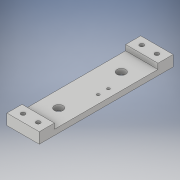
# Autodesk Inventor part: joint1_gear_holder
Saved by Autodesk Inventor 2019 (Build 230136000, 136)
## iProperties
Created: 2019-12-26
Part Number: joint1_gear_holder
Material: Типовые
Document SubType Name: Modeling
Designer: Петров Иван
Density: 1 g/cm^3
Appearance: По умолчанию
Author: Петров Иван
Autodesk Inventor part; units mm, degrees
ref_plane "YZ Plane" through (0, 0, 0) normal (1, 0, 0) x (0, 1, 0)
ref_plane "XZ Plane" through (0, 0, 0) normal (0, 1, 0) x (-1, 0, 0)
ref_plane "XY Plane" through (0, 0, 0) normal (0, 0, 1) x (1, 0, 0)
sketch "Эскиз1" plane through (0, 0, 0) normal (0, 1, 0) x (-1, 0, 0)
  line L0 (-15, 62) -> (15, 62)
  line L1 (15, 62) -> (15, -62)
  line L2 (15, -62) -> (-15, -62)
  line L3 (-15, -62) -> (-15, 62)
  line L4 (-15, 62) -> (15, -62) construction
  line L5 (15, 62) -> (-15, -62) construction
  point P0 (0, 0)
  dimension "d0" = 30
  dimension "d1" = 124
  constraints: 12 end point, 2 midpoint, 2 parallel, 1 horizontal, 1 perpendicular
  measures "d0" distance of L1.end L2.end
  measures "d1" distance of L0.end L1.end
extrude "Выдавливание1" add sketch "Эскиз1" along normal blind 5
sketch "Эскиз2" plane through (0, 5, 0) normal (0, 1, 0) x (1, 0, 0)
  line L0 (-15, -62) -> (15, -62) projected
  line L1 (15, -62) -> (15, 62) projected
  line L2 (-15, -62) -> (15, -62)
  line L3 (15, -62) -> (15, -48)
  line L4 (15, -48) -> (-15, -48)
  line L5 (-15, -48) -> (-15, -62)
  point P0 (0, 0)
  dimension "d4" = 14
  constraints: 8 end point, 2 parallel, 1 horizontal, 1 perpendicular, 1 point on line
  measures "d4" distance of L3.end L2.end
extrude "Выдавливание2" add sketch "Эскиз2" along normal blind 5
mirror "Зеркальное отражение1" about plane through (0, 0, 0) normal (0, 0, 1) of "Выдавливание2"
sketch "Эскиз3" plane through (0, 5, 0) normal (0, 1, 0) x (1, 0, 0)
  line L0 (15, 48) -> (-15, 48) projected
  line L1 (0, 48) -> (0, 29)
  circle A0 centre (0, 29) radius 4
  point P0 (0, 0)
  dimension "d7" = 19
  dimension "d8" = 8
  constraints: 2 end point, 1 centre point, 1 coincident, 1 midpoint, 1 vertical
  measures "d7" distance of L1.start L1.end
  measures "d8" diameter of A0
extrude "Выдавливание3" cut sketch "Эскиз3" against normal blind 15
mirror "Зеркальное отражение2" about plane through (0, 0, 0) normal (0, 0, 1) of "Выдавливание3"
sketch "Эскиз4" plane through (0, 0, 0) normal (0, -1, 0) x (1, 0, 0)
  line L0 (15, -62) -> (15, 62) projected
  line L1 (15, 48) -> (-15, 48) projected
  line L2 (15, 62) -> (-15, 62)
  line L3 (-15, 62) -> (-15, 48)
  line L4 (-15, 48) -> (15, 48)
  line L5 (15, 48) -> (15, 62)
  line L6 (15, 62) -> (-15, 62) projected
  line L7 (0, 62) -> (0, 55)
  line L8 (0, 55) -> (7, 55)
  circle A0 centre (7, 55) radius 1.9
  circle A1 centre (-7, 55) radius 1.9
  point P0 (0, 0)
  dimension "d11" = 7
  dimension "d12" = 7
  dimension "d13" = 3.8
  constraints: 12 end point, 2 centre point, 2 parallel, 2 perpendicular, 1 coincident, 1 horizontal, 1 midpoint, 1 symmetric about line, 1 vertical, 1 other
  measures "d11" distance of L7.start L7.end
  measures "d12" distance of L7.end L8.end
  measures "d13" diameter of A0
extrude "Выдавливание4" cut sketch "Эскиз4" against normal through all contours A0 | A1
mirror "Зеркальное отражение3" about plane through (0, 0, 0) normal (0, 0, 1) of "Выдавливание4"
sketch "Эскиз5" plane through (0, 0, 0) normal (0, -1, 0) x (1, 0, 0)
  line L0 (15.3651, -14.5668) -> (15.3651, -14.0542)
  line L1 (15.3651, -14.0542) -> (13.9311, -13.9625)
  arc A0 (13.9311, -9.7711) -> (13.9311, -13.9625) centre (14.0651, -11.8668) ccw
  line L2 (13.9311, -9.7711) -> (15.3651, -9.6794)
  line L3 (15.3651, -9.6794) -> (15.3651, -5.3911)
  arc A1 (15.3651, -5.3911) -> (15.3358, -5.3204) centre (15.2651, -5.3911) ccw
  line L4 (15.3358, -5.3204) -> (15.0115, -4.9961)
  arc A2 (14.8651, -4.6426) -> (15.0115, -4.9961) centre (15.3651, -4.6426) ccw
  line L5 (14.8651, -4.6426) -> (14.8651, 5.0332)
  arc A3 (14.8651, 5.0332) -> (14.7651, 5.1332) centre (14.7651, 5.0332) ccw
  line L6 (14.7651, 5.1332) -> (5.6151, 5.1332)
  arc A4 (5.6151, 5.1332) -> (5.5151, 5.0332) centre (5.6151, 5.0332) ccw
  line L7 (5.5151, 5.0332) -> (5.5151, 2.1074)
  arc A5 (5.3686, 1.7539) -> (5.5151, 2.1074) centre (5.0151, 2.1074) ccw
  line L8 (5.3686, 1.7539) -> (5.0444, 1.4296)
  arc A6 (5.0444, 1.4296) -> (5.0151, 1.3589) centre (5.1151, 1.3589) ccw
  line L9 (5.0151, 1.3589) -> (5.0151, -1.3926)
  arc A7 (5.0151, -1.3926) -> (5.0444, -1.4633) centre (5.1151, -1.3926) ccw
  line L10 (5.0444, -1.4633) -> (5.3686, -1.7875)
  arc A8 (5.5151, -2.1411) -> (5.3686, -1.7875) centre (5.0151, -2.1411) ccw
  line L11 (5.5151, -2.1411) -> (5.5151, -7.3926)
  arc A9 (5.3686, -7.7461) -> (5.5151, -7.3926) centre (5.0151, -7.3926) ccw
  line L12 (5.3686, -7.7461) -> (5.0444, -8.0704)
  arc A10 (5.0444, -8.0704) -> (5.0151, -8.1411) centre (5.1151, -8.1411) ccw
  line L13 (5.0151, -8.1411) -> (5.0151, -10.8926)
  arc A11 (5.0151, -10.8926) -> (5.0444, -10.9633) centre (5.1151, -10.8926) ccw
  line L14 (5.0444, -10.9633) -> (5.3686, -11.2875)
  arc A12 (5.5151, -11.6411) -> (5.3686, -11.2875) centre (5.0151, -11.6411) ccw
  line L15 (5.5151, -11.6411) -> (5.5151, -14.5668)
  arc A13 (5.5151, -14.5668) -> (5.6151, -14.6668) centre (5.6151, -14.5668) ccw
  line L16 (5.6151, -14.6668) -> (15.2651, -14.6668)
  arc A14 (15.2651, -14.6668) -> (15.3651, -14.5668) centre (15.2651, -14.5668) ccw
  circle A15 centre (7.5651, -9.5168) radius 1.25
  circle A16 centre (7.5651, -0.0168) radius 1.25
  line L17 (9.8151, 1.1565) -> (11.1151, 0.5398)
  line L18 (11.1151, 0.5398) -> (11.1151, 0.5232)
  line L19 (11.1151, 0.5232) -> (9.8151, -0.0768)
  line L20 (9.8151, -0.0768) -> (9.8151, 0.05)
  line L21 (9.8151, 0.05) -> (10.2318, 0.2422)
  line L22 (10.2318, 0.2422) -> (10.2318, 0.8315)
  line L23 (10.2318, 0.8315) -> (9.8151, 1.0292)
  line L24 (9.8151, 1.0292) -> (9.8151, 1.1565)
  spline S0 degree 3 poles (10.7516, -1.6635) (10.7604, -1.6633) (10.7779, -1.6628) (10.8035, -1.6587) (10.8283, -1.6525) (10.8522, -1.6436) (10.875, -1.6318) (10.8968, -1.6176) (10.9178, -1.6011) (10.9376, -1.582) (10.9556, -1.561) (10.9717, -1.5389) (10.985, -1.5155) (10.996, -1.4909) (11.0046, -1.4652) (11.0106, -1.4383) (11.0143, -1.4103) (11.0148, -1.3912) (11.0151, -1.3815) knots 0 0 0 0 0.061965 0.122122 0.180988 0.239933 0.299906 0.359989 0.421776 0.486576 0.551535 0.615018 0.677259 0.73973 0.80305 0.866495 0.931973 1 1 1 1
  spline S1 degree 3 poles (11.0151, -1.3815) (11.0148, -1.3713) (11.0143, -1.3513) (11.0107, -1.322) (11.0044, -1.2941) (10.9958, -1.2674) (10.9848, -1.2419) (10.9712, -1.2178) (10.9549, -1.1951) (10.9365, -1.1738) (10.916, -1.1542) (10.8931, -1.137) (10.8683, -1.1219) (10.8416, -1.1087) (10.8128, -1.098) (10.7819, -1.0899) (10.7492, -1.0834) (10.7267, -1.0813) (10.7151, -1.0802) knots 0 0 0 0 0.064439 0.126547 0.186887 0.245878 0.304041 0.362191 0.420976 0.48066 0.5406 0.600689 0.661936 0.724443 0.789038 0.856314 0.926352 1 1 1 1
  line L25 (10.7151, -1.0802) -> (10.7151, -0.9635)
  spline S2 degree 3 poles (10.7151, -0.9635) (10.7306, -0.9643) (10.761, -0.9657) (10.8053, -0.9727) (10.8477, -0.9827) (10.8877, -0.9969) (10.9258, -1.0145) (10.9619, -1.0355) (10.9957, -1.0605) (11.0269, -1.0888) (11.0556, -1.1195) (11.0803, -1.1527) (11.1013, -1.1876) (11.1188, -1.224) (11.1319, -1.2624) (11.1416, -1.3025) (11.1475, -1.3444) (11.1481, -1.3729) (11.1484, -1.3875) knots 0 0 0 0 0.068791 0.135103 0.198979 0.261904 0.323495 0.385195 0.446969 0.509765 0.572251 0.633405 0.693251 0.752583 0.812579 0.873275 0.93555 1 1 1 1
  spline S3 degree 3 poles (11.1484, -1.3875) (11.1481, -1.4017) (11.1474, -1.4297) (11.1418, -1.4706) (11.133, -1.5095) (11.1206, -1.5464) (11.104, -1.5809) (11.084, -1.6134) (11.0609, -1.6442) (11.0337, -1.6719) (11.0046, -1.6974) (10.9736, -1.7193) (10.9416, -1.7381) (10.9083, -1.7538) (10.8734, -1.7653) (10.8375, -1.7741) (10.8001, -1.779) (10.7748, -1.7798) (10.762, -1.7802) knots 0 0 0 0 0.069475 0.136517 0.200789 0.26383 0.325735 0.387291 0.449509 0.512968 0.576275 0.63758 0.697903 0.757172 0.816599 0.876653 0.93729 1 1 1 1
  spline S4 degree 3 poles (10.762, -1.7802) (10.7439, -1.7795) (10.708, -1.7783) (10.6552, -1.7676) (10.6041, -1.751) (10.563, -1.7309) (10.5298, -1.7107) (10.5026, -1.6924) (10.4732, -1.6711) (10.4418, -1.6463) (10.4082, -1.6187) (10.3723, -1.5878) (10.3346, -1.5536) (10.3089, -1.5296) (10.2956, -1.5171) knots 0 0 0 0 0.098702 0.195672 0.292422 0.391343 0.444462 0.504229 0.570352 0.642546 0.722288 0.807921 0.90047 1 1 1 1
  line L26 (10.2956, -1.5171) -> (9.9484, -1.1919)
  line L27 (9.9484, -1.1919) -> (9.9484, -1.7968)
  line L28 (9.9484, -1.7968) -> (9.8151, -1.7968)
  line L29 (9.8151, -1.7968) -> (9.8151, -0.9135)
  line L30 (9.8151, -0.9135) -> (10.3531, -1.4177)
  spline S5 degree 3 poles (10.3531, -1.4177) (10.3659, -1.4299) (10.3905, -1.4535) (10.4265, -1.4869) (10.4598, -1.5168) (10.4905, -1.5436) (10.5189, -1.5665) (10.5443, -1.5869) (10.5676, -1.6032) (10.5946, -1.621) (10.6276, -1.6381) (10.6679, -1.6529) (10.7094, -1.6619) (10.7374, -1.663) (10.7516, -1.6635) knots 0 0 0 0 0.110803 0.212829 0.306101 0.390647 0.466924 0.534481 0.593587 0.644557 0.7362 0.825024 0.911986 1 1 1 1
  line L31 (10.4651, -2.1735) -> (11.1151, -2.3068)
  line L32 (11.1151, -2.3068) -> (11.1151, -2.8402)
  line L33 (11.1151, -2.8402) -> (10.9818, -2.8402)
  line L34 (10.9818, -2.8402) -> (10.9818, -2.398)
  line L35 (10.9818, -2.398) -> (10.6398, -2.3279)
  spline S6 degree 3 poles (10.6398, -2.3279) (10.6436, -2.3417) (10.651, -2.3684) (10.6592, -2.4077) (10.6641, -2.4451) (10.6648, -2.4693) (10.6651, -2.481) knots 0 0 0 0 0.275068 0.532901 0.773973 1 1 1 1
  spline S7 degree 3 poles (10.6651, -2.481) (10.6648, -2.4956) (10.6642, -2.5241) (10.6582, -2.5659) (10.6489, -2.6057) (10.6358, -2.6436) (10.6192, -2.6796) (10.5983, -2.7133) (10.574, -2.7453) (10.546, -2.775) (10.5152, -2.802) (10.4821, -2.8257) (10.447, -2.8458) (10.4095, -2.862) (10.3702, -2.8749) (10.3285, -2.8835) (10.2849, -2.8892) (10.255, -2.8898) (10.2398, -2.8902) knots 0 0 0 0 0.065808 0.129394 0.190894 0.251281 0.310815 0.370371 0.430768 0.492881 0.555104 0.616067 0.677256 0.73826 0.800762 0.864778 0.931045 1 1 1 1
  spline S8 degree 3 poles (10.2398, -2.8902) (10.2292, -2.8899) (10.2082, -2.8894) (10.1769, -2.8869) (10.1464, -2.8821) (10.1164, -2.8757) (10.0872, -2.8673) (10.0586, -2.8572) (10.0308, -2.8448) (10.0036, -2.8312) (9.9775, -2.8158) (9.9531, -2.7988) (9.9301, -2.7809) (9.9086, -2.7615) (9.8888, -2.7407) (9.8706, -2.7185) (9.8537, -2.6952) (9.8388, -2.6705) (9.8251, -2.6448) (9.8138, -2.6178) (9.8038, -2.5901) (9.7957, -2.5614) (9.7894, -2.5317) (9.7852, -2.5008) (9.7821, -2.4691) (9.7819, -2.4476) (9.7818, -2.4368) knots 0 0 0 0 0.044014 0.087434 0.130118 0.172554 0.214555 0.256298 0.298438 0.340849 0.382715 0.423924 0.464246 0.504074 0.543862 0.583567 0.623094 0.663229 0.703551 0.743938 0.784541 0.82575 0.867757 0.910745 0.954914 1 1 1 1
  spline S9 degree 3 poles (9.7818, -2.4368) (9.782, -2.4238) (9.7825, -2.3983) (9.7878, -2.361) (9.7954, -2.3251) (9.8067, -2.2909) (9.821, -2.258) (9.839, -2.2271) (9.8594, -2.1971) (9.8835, -2.1694) (9.9099, -2.1437) (9.9385, -2.1208) (9.9688, -2.1003) (10.0011, -2.0826) (10.0352, -2.0676) (10.0713, -2.0558) (10.1091, -2.0462) (10.1352, -2.0422) (10.1484, -2.0402) knots 0 0 0 0 0.065421 0.128708 0.190236 0.250724 0.310637 0.370766 0.431615 0.493523 0.555883 0.617342 0.678668 0.740711 0.802985 0.866803 0.932347 1 1 1 1
  line L36 (10.1484, -2.0402) -> (10.1484, -2.1568)
  spline S10 degree 3 poles (10.1484, -2.1568) (10.136, -2.1597) (10.1122, -2.1652) (10.0787, -2.1773) (10.0489, -2.1921) (10.0223, -2.2097) (9.9991, -2.2307) (9.9785, -2.2547) (9.9598, -2.2816) (9.9443, -2.3114) (9.9311, -2.3429) (9.9222, -2.3759) (9.916, -2.4095) (9.9154, -2.4321) (9.9151, -2.4435) knots 0 0 0 0 0.094687 0.181994 0.264377 0.34218 0.418618 0.496509 0.577369 0.661511 0.746733 0.831258 0.915206 1 1 1 1
  spline S11 degree 3 poles (9.9151, -2.4435) (9.9154, -2.4547) (9.916, -2.4766) (9.9206, -2.5088) (9.9277, -2.54) (9.9384, -2.5697) (9.9513, -2.5985) (9.9679, -2.6257) (9.9871, -2.652) (10.0089, -2.6767) (10.0331, -2.6993) (10.0589, -2.7192) (10.0864, -2.7359) (10.1152, -2.7499) (10.1455, -2.7605) (10.1773, -2.7681) (10.2105, -2.7726) (10.2332, -2.7732) (10.2448, -2.7735) knots 0 0 0 0 0.064207 0.126425 0.18768 0.248216 0.308305 0.369661 0.431699 0.495947 0.559758 0.622295 0.683911 0.745092 0.80674 0.869087 0.93329 1 1 1 1
  spline S12 degree 3 poles (10.2448, -2.7735) (10.2552, -2.7733) (10.2756, -2.7728) (10.3055, -2.7689) (10.3337, -2.7621) (10.3605, -2.7526) (10.3859, -2.7406) (10.4098, -2.726) (10.432, -2.7084) (10.4524, -2.6883) (10.4713, -2.6663) (10.4874, -2.642) (10.501, -2.6159) (10.5127, -2.5883) (10.521, -2.5586) (10.5274, -2.5274) (10.531, -2.4942) (10.5315, -2.4716) (10.5318, -2.46) knots 0 0 0 0 0.065351 0.127916 0.18836 0.247216 0.30563 0.36377 0.422661 0.482687 0.5433 0.604118 0.664965 0.727413 0.791468 0.858055 0.927037 1 1 1 1
  spline S13 degree 3 poles (10.5318, -2.46) (10.5315, -2.4499) (10.5311, -2.4291) (10.5278, -2.3972) (10.5225, -2.3636) (10.5153, -2.3286) (10.5057, -2.292) (10.4943, -2.2538) (10.4807, -2.2141) (10.4704, -2.1873) (10.4651, -2.1735) knots 0 0 0 0 0.102203 0.211023 0.3251 0.446502 0.573788 0.708901 0.850358 1 1 1 1
  line L37 (9.8151, -5.6202) -> (11.1151, -6.2368)
  line L38 (11.1151, -6.2368) -> (11.1151, -6.2535)
  line L39 (11.1151, -6.2535) -> (9.8151, -6.8535)
  line L40 (9.8151, -6.8535) -> (9.8151, -6.7267)
  line L41 (9.8151, -6.7267) -> (10.2318, -6.5345)
  line L42 (10.2318, -6.5345) -> (10.2318, -5.9452)
  line L43 (10.2318, -5.9452) -> (9.8151, -5.7475)
  line L44 (9.8151, -5.7475) -> (9.8151, -5.6202)
  spline S14 degree 3 poles (10.4726, -7.1302) (10.496, -7.1307) (10.542, -7.1319) (10.6096, -7.1415) (10.6742, -7.1571) (10.736, -7.1791) (10.7951, -7.2071) (10.8511, -7.2416) (10.9044, -7.2824) (10.9542, -7.329) (10.9997, -7.3801) (11.0397, -7.4348) (11.0731, -7.493) (11.1009, -7.5541) (11.1223, -7.6186) (11.1373, -7.6862) (11.1467, -7.7569) (11.1478, -7.8051) (11.1484, -7.8296) knots 0 0 0 0 0.064558 0.127014 0.187955 0.248014 0.307748 0.368235 0.42947 0.492743 0.556258 0.618217 0.679655 0.741246 0.803415 0.866815 0.932328 1 1 1 1
  spline S15 degree 3 poles (11.1484, -7.8296) (11.1482, -7.8446) (11.1479, -7.8741) (11.1444, -7.9179) (11.1387, -7.9605) (11.1308, -8.0019) (11.1211, -8.0424) (11.1084, -8.0817) (11.0939, -8.12) (11.0772, -8.1571) (11.0585, -8.1927) (11.0379, -8.2269) (11.0155, -8.2594) (10.9915, -8.2904) (10.9653, -8.3194) (10.9378, -8.3473) (10.908, -8.373) (10.8871, -8.3889) (10.8766, -8.3968) knots 0 0 0 0 0.068548 0.135683 0.201215 0.265682 0.329267 0.392395 0.45507 0.517127 0.57879 0.63974 0.700192 0.759806 0.819628 0.879355 0.939512 1 1 1 1
  line L45 (10.8766, -8.3968) -> (10.7984, -8.2947)
  spline S16 degree 3 poles (10.7984, -8.2947) (10.8071, -8.2875) (10.8243, -8.273) (10.8486, -8.2497) (10.8712, -8.2255) (10.8925, -8.2002) (10.9116, -8.1736) (10.9295, -8.1462) (10.9456, -8.1175) (10.9651, -8.0778) (10.9854, -8.026) (11.0025, -7.9607) (11.0133, -7.8925) (11.0145, -7.846) (11.0151, -7.8223) knots 0 0 0 0 0.063163 0.125475 0.187121 0.248294 0.309295 0.36985 0.430973 0.492456 0.616148 0.740844 0.868183 1 1 1 1
  spline S17 degree 3 poles (11.0151, -7.8223) (11.0149, -7.8093) (11.0146, -7.7834) (11.0107, -7.7449) (11.0052, -7.7071) (10.9969, -7.6701) (10.9866, -7.6338) (10.9741, -7.5981) (10.9588, -7.5635) (10.9418, -7.5295) (10.9226, -7.4969) (10.9017, -7.466) (10.8793, -7.437) (10.8553, -7.4099) (10.8298, -7.3846) (10.8025, -7.3613) (10.7736, -7.34) (10.7434, -7.3204) (10.712, -7.3029) (10.6793, -7.2882) (10.6458, -7.2752) (10.6112, -7.2649) (10.5757, -7.2568) (10.5393, -7.2512) (10.5019, -7.2473) (10.4766, -7.247) (10.4638, -7.2468) knots 0 0 0 0 0.043955 0.087502 0.130463 0.172752 0.215403 0.25765 0.300153 0.343121 0.385925 0.427686 0.468818 0.509492 0.549883 0.58998 0.630405 0.670869 0.711384 0.751627 0.791776 0.832459 0.873319 0.914543 0.956924 1 1 1 1
  spline S18 degree 3 poles (10.4638, -7.2468) (10.4446, -7.2473) (10.4069, -7.2482) (10.3516, -7.2564) (10.2987, -7.2689) (10.2484, -7.2875) (10.2001, -7.3105) (10.1547, -7.3396) (10.1115, -7.3732) (10.0714, -7.412) (10.0348, -7.4544) (10.0026, -7.5) (9.9758, -7.5486) (9.9534, -7.5996) (9.9362, -7.6535) (9.9241, -7.7101) (9.9162, -7.7694) (9.9155, -7.8098) (9.9151, -7.8304) knots 0 0 0 0 0.064323 0.12629 0.186726 0.246146 0.305576 0.365429 0.426326 0.48884 0.551725 0.613919 0.675484 0.737334 0.800229 0.864502 0.931041 1 1 1 1
  spline S19 degree 3 poles (9.9151, -7.8304) (9.9157, -7.8531) (9.917, -7.8978) (9.9274, -7.9633) (9.9444, -8.026) (9.9681, -8.0859) (9.999, -8.1429) (10.0364, -8.197) (10.0807, -8.2482) (10.1145, -8.279) (10.1318, -8.2947) knots 0 0 0 0 0.128515 0.252949 0.374755 0.49594 0.617181 0.740909 0.867811 1 1 1 1
  line L46 (10.1318, -8.2947) -> (10.0544, -8.3968)
  spline S20 degree 3 poles (10.0544, -8.3968) (10.0438, -8.3886) (10.0227, -8.3722) (9.9929, -8.3457) (9.9648, -8.3177) (9.9388, -8.2881) (9.9142, -8.2573) (9.8918, -8.2245) (9.8713, -8.1904) (9.8525, -8.155) (9.8358, -8.1183) (9.8215, -8.0804) (9.8092, -8.0415) (9.7991, -8.0015) (9.7912, -7.9604) (9.7859, -7.9183) (9.7823, -7.8751) (9.7819, -7.846) (9.7818, -7.8312) knots 0 0 0 0 0.061674 0.123053 0.183475 0.243727 0.304279 0.364863 0.425946 0.487391 0.54922 0.611144 0.673529 0.736961 0.800785 0.866013 0.932101 1 1 1 1
  spline S21 degree 3 poles (9.7818, -7.8312) (9.7819, -7.8172) (9.7821, -7.7896) (9.7852, -7.7488) (9.7894, -7.709) (9.7958, -7.6705) (9.8034, -7.6329) (9.8135, -7.5967) (9.8249, -7.5614) (9.8382, -7.5272) (9.8532, -7.4942) (9.8703, -7.4623) (9.8891, -7.4316) (9.9093, -7.4018) (9.9316, -7.3733) (9.9556, -7.346) (9.9813, -7.3196) (9.9998, -7.3032) (10.0091, -7.295) knots 0 0 0 0 0.069663 0.13775 0.203917 0.26878 0.332414 0.394754 0.45618 0.516996 0.577396 0.637198 0.696999 0.756756 0.816554 0.876948 0.938132 1 1 1 1
  spline S22 degree 3 poles (10.0091, -7.295) (10.0253, -7.2818) (10.0574, -7.2557) (10.1095, -7.2222) (10.1639, -7.1935) (10.2209, -7.1704) (10.2804, -7.1523) (10.3423, -7.1397) (10.4066, -7.1316) (10.4504, -7.1306) (10.4726, -7.1302) knots 0 0 0 0 0.124329 0.247156 0.36878 0.490734 0.613614 0.738958 0.867311 1 1 1 1
  line L47 (11.0651, -10.2028) -> (11.0651, -9.99)
  line L48 (9.9651, -9.8025) -> (11.0651, -10.2028)
  line L49 (9.9651, -10.3025) -> (9.9651, -9.8025)
  line L50 (11.0651, -10.7028) -> (9.9651, -10.3025)
  line L51 (11.0651, -10.9157) -> (11.0651, -10.7028)
  line L52 (9.9651, -10.5153) -> (11.0651, -10.9157)
  line L53 (9.9651, -10.7153) -> (9.9651, -10.5153)
  line L54 (9.7651, -10.6425) -> (9.9651, -10.7153)
  line L55 (9.7651, -9.5168) -> (9.7651, -10.6425)
  line L56 (11.0651, -9.99) -> (9.7651, -9.5168)
  line L57 (9.8151, -4.8268) -> (9.8151, -4.8102)
  line L58 (9.8151, -4.8102) -> (11.1151, -4.2602)
  line L59 (11.1151, -4.2602) -> (11.1151, -4.3852)
  line L60 (11.1151, -4.3852) -> (10.0906, -4.8185)
  line L61 (10.0906, -4.8185) -> (11.1151, -5.2518)
  line L62 (11.1151, -5.2518) -> (11.1151, -5.3768)
  line L63 (11.1151, -5.3768) -> (9.8151, -4.8268)
  spline S23 degree 3 poles (10.4646, -4.0168) (10.4447, -4.0166) (10.406, -4.0161) (10.3493, -4.0137) (10.2958, -4.0089) (10.2454, -4.0028) (10.1982, -3.9945) (10.1541, -3.9842) (10.1129, -3.9729) (10.0749, -3.9588) (10.0396, -3.9434) (10.0067, -3.9267) (9.9758, -3.9088) (9.9472, -3.8892) (9.9207, -3.8684) (9.8967, -3.8459) (9.8748, -3.8222) (9.8552, -3.7972) (9.8381, -3.771) (9.8228, -3.7443) (9.8104, -3.7165) (9.7998, -3.6883) (9.7917, -3.6593) (9.7861, -3.6295) (9.7822, -3.5991) (9.7819, -3.5785) (9.7818, -3.5681) knots 0 0 0 0 0.065063 0.126773 0.185516 0.240765 0.29298 0.34225 0.388919 0.432776 0.474628 0.514775 0.553606 0.591426 0.628028 0.663804 0.698984 0.733591 0.767628 0.801208 0.834264 0.866981 0.89972 0.932702 0.966176 1 1 1 1
  spline S24 degree 3 poles (9.7818, -3.5681) (9.7819, -3.5579) (9.7823, -3.5377) (9.7858, -3.5077) (9.7915, -3.4786) (9.7994, -3.4503) (9.8092, -3.4225) (9.8219, -3.3958) (9.8365, -3.3697) (9.8531, -3.3443) (9.8722, -3.3201) (9.8933, -3.2971) (9.9169, -3.2757) (9.9427, -3.2558) (9.9704, -3.2368) (10.0005, -3.2194) (10.0328, -3.2033) (10.0674, -3.1886) (10.105, -3.1755) (10.1459, -3.164) (10.1905, -3.1549) (10.2385, -3.1471) (10.29, -3.1408) (10.3451, -3.1365) (10.4037, -3.1339) (10.4439, -3.1336) (10.4646, -3.1335) knots 0 0 0 0 0.033787 0.066622 0.099285 0.131361 0.163585 0.196104 0.228902 0.262158 0.295991 0.330218 0.36506 0.400951 0.43762 0.475708 0.515381 0.556414 0.599765 0.646424 0.696431 0.749782 0.806573 0.867436 0.931887 1 1 1 1
  spline S25 degree 3 poles (10.4646, -3.1335) (10.4854, -3.1336) (10.5259, -3.1339) (10.5849, -3.1365) (10.6402, -3.1409) (10.6919, -3.1469) (10.7399, -3.1541) (10.7842, -3.1639) (10.8249, -3.175) (10.8622, -3.1878) (10.8966, -3.2023) (10.9287, -3.218) (10.9585, -3.2357) (10.9864, -3.2543) (11.012, -3.2745) (11.0356, -3.2958) (11.0568, -3.3189) (11.076, -3.3432) (11.0929, -3.3689) (11.1078, -3.3951) (11.1205, -3.4221) (11.1305, -3.45) (11.1387, -3.4785) (11.1444, -3.5077) (11.1479, -3.5377) (11.1483, -3.5579) (11.1484, -3.5681) knots 0 0 0 0 0.068595 0.133246 0.194313 0.251279 0.304513 0.354235 0.400481 0.443411 0.484015 0.523252 0.561042 0.5979 0.633518 0.668314 0.702496 0.736685 0.770293 0.803437 0.835913 0.86846 0.900847 0.933467 0.966258 1 1 1 1
  spline S26 degree 3 poles (11.1484, -3.5681) (11.1482, -3.5785) (11.1479, -3.599) (11.1444, -3.6294) (11.1387, -3.6591) (11.1305, -3.688) (11.1204, -3.7163) (11.1078, -3.7437) (11.093, -3.7705) (11.0757, -3.7963) (11.0564, -3.8213) (11.0346, -3.8448) (11.0105, -3.867) (10.9843, -3.8881) (10.9556, -3.9074) (10.9248, -3.9258) (10.8915, -3.9423) (10.8562, -3.9582) (10.8178, -3.9719) (10.7767, -3.9842) (10.7323, -3.9942) (10.6848, -4.0025) (10.6341, -4.009) (10.5804, -4.0136) (10.5235, -4.0161) (10.4845, -4.0166) (10.4646, -4.0168) knots 0 0 0 0 0.033788 0.067194 0.099862 0.132567 0.165151 0.197913 0.231319 0.265083 0.299255 0.334399 0.369943 0.406284 0.444064 0.482998 0.523354 0.565537 0.609613 0.656391 0.705885 0.758325 0.813832 0.872795 0.934722 1 1 1 1
  line L64 (10.4651, 2.1332) -> (11.1151, 1.9998)
  line L65 (11.1151, 1.9998) -> (11.1151, 1.4665)
  line L66 (11.1151, 1.4665) -> (10.9818, 1.4665)
  line L67 (10.9818, 1.4665) -> (10.9818, 1.9087)
  line L68 (10.9818, 1.9087) -> (10.6398, 1.9787)
  spline S27 degree 3 poles (10.6398, 1.9787) (10.6436, 1.965) (10.651, 1.9383) (10.6592, 1.899) (10.6641, 1.8616) (10.6648, 1.8374) (10.6651, 1.8256) knots 0 0 0 0 0.275068 0.532901 0.773973 1 1 1 1
  spline S28 degree 3 poles (10.6651, 1.8256) (10.6648, 1.8111) (10.6642, 1.7826) (10.6582, 1.7408) (10.6489, 1.7009) (10.6358, 1.663) (10.6192, 1.6271) (10.5983, 1.5933) (10.574, 1.5613) (10.546, 1.5316) (10.5152, 1.5047) (10.4821, 1.481) (10.447, 1.4609) (10.4095, 1.4447) (10.3702, 1.4318) (10.3285, 1.4232) (10.2849, 1.4175) (10.255, 1.4168) (10.2398, 1.4165) knots 0 0 0 0 0.065808 0.129394 0.190894 0.251281 0.310815 0.370371 0.430768 0.492881 0.555104 0.616067 0.677256 0.73826 0.800762 0.864778 0.931045 1 1 1 1
  spline S29 degree 3 poles (10.2398, 1.4165) (10.2292, 1.4168) (10.2082, 1.4172) (10.1769, 1.4197) (10.1464, 1.4245) (10.1164, 1.431) (10.0872, 1.4394) (10.0586, 1.4495) (10.0308, 1.4619) (10.0036, 1.4755) (9.9775, 1.4908) (9.9531, 1.5078) (9.9301, 1.5258) (9.9086, 1.5451) (9.8888, 1.566) (9.8706, 1.5882) (9.8537, 1.6115) (9.8388, 1.6362) (9.8251, 1.6619) (9.8138, 1.6889) (9.8038, 1.7165) (9.7957, 1.7453) (9.7894, 1.775) (9.7852, 1.8058) (9.7821, 1.8375) (9.7819, 1.859) (9.7818, 1.8699) knots 0 0 0 0 0.044014 0.087434 0.130118 0.172554 0.214555 0.256298 0.298438 0.340849 0.382715 0.423924 0.464246 0.504074 0.543862 0.583567 0.623094 0.663229 0.703551 0.743938 0.784541 0.82575 0.867757 0.910745 0.954914 1 1 1 1
  spline S30 degree 3 poles (9.7818, 1.8699) (9.782, 1.8828) (9.7825, 1.9083) (9.7878, 1.9457) (9.7954, 1.9816) (9.8067, 2.0158) (9.821, 2.0486) (9.839, 2.0796) (9.8594, 2.1096) (9.8835, 2.1372) (9.9099, 2.1629) (9.9385, 2.1859) (9.9688, 2.2064) (10.0011, 2.224) (10.0352, 2.2391) (10.0713, 2.2509) (10.1091, 2.2604) (10.1352, 2.2645) (10.1484, 2.2665) knots 0 0 0 0 0.065421 0.128708 0.190236 0.250724 0.310637 0.370766 0.431615 0.493523 0.555883 0.617342 0.678668 0.740711 0.802985 0.866803 0.932347 1 1 1 1
  line L69 (10.1484, 2.2665) -> (10.1484, 2.1498)
  spline S31 degree 3 poles (10.1484, 2.1498) (10.136, 2.147) (10.1122, 2.1415) (10.0787, 2.1293) (10.0489, 2.1145) (10.0223, 2.0969) (9.9991, 2.0759) (9.9785, 2.052) (9.9598, 2.0251) (9.9443, 1.9952) (9.9311, 1.9637) (9.9222, 1.9307) (9.916, 1.8972) (9.9154, 1.8745) (9.9151, 1.8631) knots 0 0 0 0 0.094687 0.181994 0.264377 0.34218 0.418618 0.496509 0.577369 0.661511 0.746733 0.831258 0.915206 1 1 1 1
  spline S32 degree 3 poles (9.9151, 1.8631) (9.9154, 1.852) (9.916, 1.8301) (9.9206, 1.7978) (9.9277, 1.7667) (9.9384, 1.737) (9.9513, 1.7082) (9.9679, 1.681) (9.9871, 1.6547) (10.0089, 1.63) (10.0331, 1.6074) (10.0589, 1.5874) (10.0864, 1.5708) (10.1152, 1.5568) (10.1455, 1.5461) (10.1773, 1.5386) (10.2105, 1.5341) (10.2332, 1.5335) (10.2448, 1.5332) knots 0 0 0 0 0.064207 0.126425 0.18768 0.248216 0.308305 0.369661 0.431699 0.495947 0.559758 0.622295 0.683911 0.745092 0.80674 0.869087 0.93329 1 1 1 1
  spline S33 degree 3 poles (10.2448, 1.5332) (10.2552, 1.5334) (10.2756, 1.5339) (10.3055, 1.5378) (10.3337, 1.5446) (10.3605, 1.5541) (10.3859, 1.566) (10.4098, 1.5807) (10.432, 1.5983) (10.4524, 1.6184) (10.4713, 1.6404) (10.4874, 1.6647) (10.501, 1.6908) (10.5127, 1.7184) (10.521, 1.7481) (10.5274, 1.7793) (10.531, 1.8124) (10.5315, 1.8351) (10.5318, 1.8467) knots 0 0 0 0 0.065351 0.127916 0.18836 0.247216 0.30563 0.36377 0.422661 0.482687 0.5433 0.604118 0.664965 0.727413 0.791468 0.858055 0.927037 1 1 1 1
  spline S34 degree 3 poles (10.5318, 1.8467) (10.5315, 1.8568) (10.5311, 1.8776) (10.5278, 1.9095) (10.5225, 1.943) (10.5153, 1.9781) (10.5057, 2.0147) (10.4943, 2.0529) (10.4807, 2.0926) (10.4704, 2.1194) (10.4651, 2.1332) knots 0 0 0 0 0.102203 0.211023 0.3251 0.446502 0.573788 0.708901 0.850358 1 1 1 1
  point P0 (0, 0)
  point P1 (7.5651, -9.5168)
  constraints: 140 end point, 30 point on circle, 17 centre point, 72 other
extrude "Выдавливание5" cut sketch "Эскиз5" against normal through all contours A15 | A16
